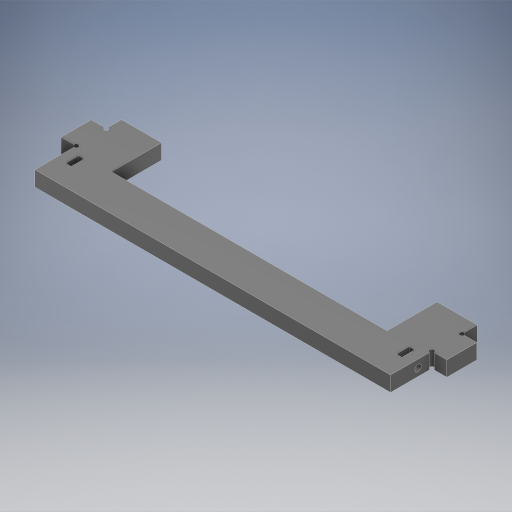
# Autodesk Inventor part: battery backplate
Saved by Autodesk Inventor 2024 (Build 280153000, 153)
## iProperties
Created: 2024-09-04
Part Number: battery backplate
Material: PMMA 플라스틱
Document SubType Name: Modeling
Designer: msi
Density: 1.188 g/cm^3
Appearance: 매끄러움 - 검은색
Author: msi
Autodesk Inventor part; units mm, degrees
ref_plane "우측면도" through (0, 0, 0) normal (1, 0, 0) x (0, 1, 0)
ref_plane "평면도" through (0, 0, 0) normal (0, 1, 0) x (-1, 0, 0)
ref_plane "정면도" through (0, 0, 0) normal (0, 0, 1) x (1, 0, 0)
sketch "스케치1" plane through (0, 0, 0) normal (0, 1, 0) x (-1, 0, 0)
  line L0 (-71, 24.6) -> (71, 24.6)
  line L1 (71, 24.6) -> (71, -10)
  line L2 (-71, -10) -> (-71, 24.6)
  line L3 (-71, 24.6) -> (71, -24.6) construction
  line L4 (71, 24.6) -> (-71, -24.6) construction
  line L5 (-71, 8.1) -> (-77, 8.1)
  line L6 (-77, 8.1) -> (-77, -3.9)
  line L7 (-77, -3.9) -> (-71, -3.9)
  line L8 (-71, -3.9) -> (-71, 8.1)
  line L9 (71, 8.1) -> (77, 8.1)
  line L10 (77, 8.1) -> (77, -3.9)
  line L11 (77, -3.9) -> (71, -3.9)
  line L12 (71, -3.9) -> (71, 8.1)
  line L13 (27.5, 10) -> (-27.5, 10)
  line L14 (-27.5, 10) -> (-27.5, -10)
  line L15 (-27.5, -10) -> (27.5, -10)
  line L16 (27.5, -10) -> (27.5, 10)
  line L17 (27.5, 10) -> (-27.5, -10) construction
  line L18 (-27.5, 10) -> (27.5, -10) construction
  line L19 (27.5, -10) -> (71, -10)
  line L20 (-27.5, -10) -> (-71, -10)
  line L21 (71, -24.6) -> (67.65, -24.6)
  line L22 (-67.65, -24.6) -> (-71, -24.6)
  point P0 (0, 0)
  dimension "d0" = 142
  dimension "d1" = 49.2
  dimension "d2" = 6
  dimension "d3" = 12
  dimension "d4" = 6
  dimension "d5" = 55
  dimension "d6" = 20
  constraints: 46 end point, 9 parallel, 7 point on line, 4 horizontal, 4 midpoint, 4 perpendicular
  measures "d0" distance of L3.end L4.end
  measures "d1" distance of L0.end L3.end
  measures "d2" distance of L7.end L6.end
  measures "d3" distance of L6.end L5.end
  measures "d4" distance of L10.end L11.end
  measures "d5" distance of L15.end L14.end
  measures "d6" distance of L14.end L13.end
extrude "돌출2" add sketch "스케치1" along normal blind 6 contours L0 L1 L19 L16 L13 L14 L20 L2 | L2 L7 L6 L5 | L9 L10 L11 L1
sketch "스케치2" plane through (0, 6, 0) normal (0, 1, 0) x (1, 0, 0)
  line L0 (-50, 10) -> (50, 10)
  line L1 (50, 10) -> (50, -10)
  line L2 (50, -10) -> (-50, -10)
  line L3 (-50, -10) -> (-50, 10)
  line L4 (-50, 10) -> (50, -10) construction
  line L5 (50, 10) -> (-50, -10) construction
  point P0 (0, 0)
  dimension "d11" = 100
  dimension "d12" = 20
  constraints: 12 end point, 2 midpoint, 2 parallel, 1 horizontal, 1 perpendicular
  measures "d11" distance of L1.end L2.end
  measures "d12" distance of L0.end L1.end
extrude "돌출3" cut sketch "스케치2" against normal blind 6
sketch "스케치3" plane through (71, 0, 24.6) normal (1, 0, 0) x (0, 0, -1)
  circle A0 centre (11, 2.9) radius 1.35 projected
  circle A1 centre (11, 2.9) radius 1.35
  point P0 (24.6, 0)
  constraints: 1 centre point, 1 coincident, 1 concentric
extrude "돌출4" cut sketch "스케치3" against normal blind 15
sketch "스케치4" plane through (-71, 0, 8.1) normal (-1, 0, 0) x (0, 0, 1)
  circle A0 centre (5.5, 2.9) radius 1.35 projected
  circle A1 centre (5.5, 2.9) radius 1.35
  point P0 (-8.1, 0)
  constraints: 1 centre point, 1 coincident, 1 concentric
extrude "돌출5" cut sketch "스케치4" against normal blind 15
sketch "스케치5" plane through (0, 6, 0) normal (0, 1, 0) x (1, 0, 0)
  line L0 (71, -12.25) -> (56, -12.25) projected
  line L1 (71, -14.95) -> (56, -14.95) projected
  line L2 (-71, -12.25) -> (-56, -12.25) projected
  line L3 (-71, -14.95) -> (-56, -14.95) projected
  line L4 (-66, -12.25) -> (-66, -14.95)
  line L5 (66, -12.25) -> (66, -14.95)
  line L6 (-67.1, -16.2) -> (-64.9, -16.2)
  line L7 (-64.9, -16.2) -> (-64.9, -11)
  line L8 (-64.9, -11) -> (-67.1, -11)
  line L9 (-67.1, -11) -> (-67.1, -16.2)
  line L10 (-67.1, -16.2) -> (-64.9, -11) construction
  line L11 (-64.9, -16.2) -> (-67.1, -11) construction
  line L12 (67.1, -16.2) -> (64.9, -16.2)
  line L13 (64.9, -16.2) -> (64.9, -11)
  line L14 (64.9, -11) -> (67.1, -11)
  line L15 (67.1, -11) -> (67.1, -16.2)
  line L16 (67.1, -16.2) -> (64.9, -11) construction
  line L17 (64.9, -16.2) -> (67.1, -11) construction
  point P0 (0, 0)
  point P1 (-66, -13.6)
  point P2 (66, -13.6)
  dimension "d19" = 2.2
  dimension "d20" = 5.2
  dimension "d21" = 2.2
  dimension "d22" = 5.2
  constraints: 28 end point, 6 midpoint, 4 parallel, 4 perpendicular, 4 point on line, 2 horizontal
  measures "d19" distance of L8.end L7.end
  measures "d20" distance of L7.end L6.end
  measures "d21" distance of L13.end L14.end
  measures "d22" distance of L12.end L13.end
extrude "돌출6" cut sketch "스케치5" against normal blind 15
sketch "스케치6" plane through (0, 6, 0) normal (0, 1, 0) x (1, 0, 0)
  line L0 (67.1, -11) -> (67.1, -16.2) projected
  line L1 (67.1, -16.2) -> (64.9, -16.2) projected
  line L2 (64.9, -16.2) -> (64.9, -11) projected
  line L3 (64.9, -11) -> (67.1, -11) projected
  line L4 (-67.1, -16.2) -> (-67.1, -11) projected
  line L5 (-67.1, -11) -> (-64.9, -11) projected
  line L6 (-64.9, -11) -> (-64.9, -16.2) projected
  line L7 (-64.9, -16.2) -> (-67.1, -16.2) projected
  line L8 (-50, -10) -> (-50, 10) projected
  line L9 (-50, 10) -> (-71, 10) projected
  line L10 (-71, 10) -> (-71, 3.9) projected
  line L11 (-71, 3.9) -> (-77, 3.9) projected
  line L12 (-77, 3.9) -> (-77, -8.1) projected
  line L13 (-77, -8.1) -> (-71, -8.1) projected
  line L14 (-71, -8.1) -> (-71, -24.6) projected
  line L15 (-71, -24.6) -> (71, -24.6) projected
  line L16 (71, -24.6) -> (71, -8.1) projected
  line L17 (71, -8.1) -> (77, -8.1) projected
  line L18 (77, -8.1) -> (77, 3.9) projected
  line L19 (77, 3.9) -> (71, 3.9) projected
  line L20 (71, 3.9) -> (71, 10) projected
  line L21 (71, 10) -> (50, 10) projected
  line L22 (50, 10) -> (50, -10) projected
  line L23 (50, -10) -> (-50, -10) projected
  line L24 (-55, -10) -> (55, -10)
  line L25 (55, -10) -> (55, 10)
  line L26 (55, 10) -> (-55, 10)
  line L27 (-55, 10) -> (-55, -10)
  line L28 (-55, -10) -> (55, 10) construction
  line L29 (55, -10) -> (-55, 10) construction
  point P0 (0, 0)
  dimension "d25" = 110
  constraints: 12 end point, 2 midpoint, 2 parallel, 1 horizontal, 1 perpendicular, 1 point on line
  measures "d25" distance of L26.end L25.end
extrude "돌출8" cut sketch "스케치6" against normal blind 10 contours L24 L27 L9 L8 | L22 L21 L25 L24
sketch "스케치7" plane through (0, 6, 0) normal (0, 1, 0) x (1, 0, 0)
  line L0 (-67.1, -16.2) -> (-67.1, -11) projected
  line L1 (-67.1, -11) -> (-64.9, -11) projected
  line L2 (-64.9, -11) -> (-64.9, -16.2) projected
  line L3 (-64.9, -16.2) -> (-67.1, -16.2) projected
  line L4 (67.1, -11) -> (67.1, -16.2) projected
  line L5 (67.1, -16.2) -> (64.9, -16.2) projected
  line L6 (64.9, -16.2) -> (64.9, -11) projected
  line L7 (64.9, -11) -> (67.1, -11) projected
  line L8 (55, 10) -> (55, -10) projected
  line L9 (55, -10) -> (-55, -10) projected
  line L10 (-55, -10) -> (-55, 10) projected
  line L11 (-55, 10) -> (-71, 10) projected
  line L12 (-71, 10) -> (-71, 3.9) projected
  line L13 (-71, 3.9) -> (-77, 3.9) projected
  line L14 (-77, 3.9) -> (-77, -8.1) projected
  line L15 (-77, -8.1) -> (-71, -8.1) projected
  line L16 (-71, -8.1) -> (-71, -24.6) projected
  line L17 (-71, -24.6) -> (71, -24.6) projected
  line L18 (71, -24.6) -> (71, -8.1) projected
  line L19 (71, -8.1) -> (77, -8.1) projected
  line L20 (77, -8.1) -> (77, 3.9) projected
  line L21 (77, 3.9) -> (71, 3.9) projected
  line L22 (71, 3.9) -> (71, 10) projected
  line L23 (71, 10) -> (55, 10) projected
  circle A0 centre (-71, 3.9) radius 1
  circle A1 centre (-71, -8.1) radius 1
  circle A2 centre (71, -8.1) radius 1
  circle A3 centre (71, 3.9) radius 1
  point P0 (0, 0)
  point P1 (72, -8.1)
  point P2 (71, -9.1)
  point P3 (71, 4.9)
  point P4 (72, 3.9)
  point P5 (-71, 4.9)
  point P6 (-72, 3.9)
  point P7 (-71, -9.1)
  point P8 (-72, -8.1)
  dimension "d30" = 2
  dimension "d31" = 2
  dimension "d32" = 2
  dimension "d33" = 2
  constraints: 4 centre point, 4 coincident
  measures "d30" diameter of A0
  measures "d31" diameter of A1
  measures "d32" diameter of A2
  measures "d33" diameter of A3
extrude "돌출9" cut sketch "스케치7" against normal blind 10 contours L22 L21 A3 | A0 L13 L12 | L19 L18 A2 | A1 L16 L15 picked at (71.1358, 3.2525) picked at (-71.657, 3.8202) picked at (71.1358, -7.4525) picked at (-71, -7.4382)
